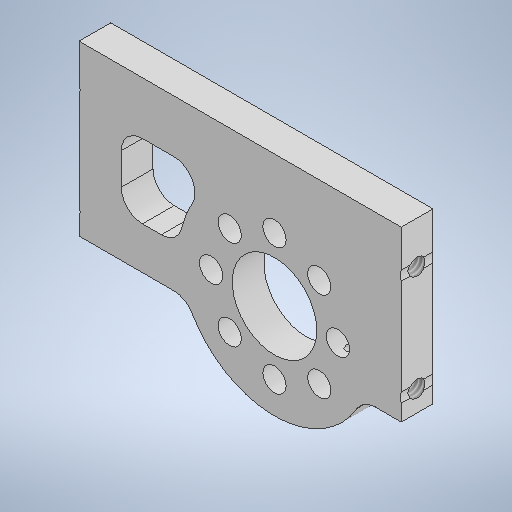
# Autodesk Inventor part: kosipich
Saved by Autodesk Inventor 2025.1 (Build 291241000, 241)
## iProperties
Created: 2024-08-31
Part Number: kosipich
Material: 一般
Document SubType Name: Modeling
Designer: right
Density: 1 g/cm^3
Appearance: 既定
Author: right
Autodesk Inventor part; units mm, degrees
ref_plane "YZ Plane" through (0, 0, 0) normal (1, 0, 0) x (0, 1, 0)
ref_plane "XZ Plane" through (0, 0, 0) normal (0, 1, 0) x (-1, 0, 0)
ref_plane "XY Plane" through (0, 0, 0) normal (0, 0, 1) x (1, 0, 0)
sketch "スケッチ1" plane through (0, 0, 0) normal (0, 0, 1) x (1, 0, 0)
  line L0 (-15.25, -12.5) -> (15.25, -12.5)
  line L1 (15.25, -12.5) -> (15.25, 12.5)
  line L2 (15.25, 12.5) -> (-15.25, 12.5)
  line L3 (-15.25, 12.5) -> (-15.25, -12.5)
  line L4 (-15.25, -12.5) -> (15.25, 12.5) construction
  line L5 (15.25, -12.5) -> (-15.25, 12.5) construction
  line L6 (-16.75, -5) -> (16.75, -5)
  line L7 (16.75, -5) -> (16.75, 5)
  line L8 (16.75, 5) -> (-16.75, 5)
  line L9 (-16.75, 5) -> (-16.75, -5)
  line L10 (-16.75, -5) -> (16.75, 5) construction
  line L11 (16.75, -5) -> (-16.75, 5) construction
  circle A0 centre (-15.25, 6.1) radius 1.1
  line L12 (0, 5) -> (0, 0) construction
  line L13 (-16.75, 0) -> (0, 0) construction
  circle A1 centre (-15.25, -6.1) radius 1.1
  circle A2 centre (15.25, 6.1) radius 1.1
  circle A3 centre (15.25, -6.1) radius 1.1
  point P0 (-15.25, -5)
  point P1 (-15.25, -7.2)
  point P2 (15.25, -7.2)
  point P3 (15.25, -5)
  point P4 (15.25, 5)
  point P5 (15.25, 7.2)
  point P6 (-15.25, 7.2)
  point P7 (-15.25, 5)
  dimension "d0" = 30.5
  dimension "d1" = 25
  dimension "d2" = 1.5
  dimension "d3" = 10
  dimension "d4" = 2.2
  constraints: 28 end point, 6 midpoint, 4 centre point, 4 parallel, 3 symmetric about line, 2 horizontal, 2 perpendicular, 1 point on line, 1 tangent, 1 vertical, 3 other
  measures "d0" distance of L2.end L1.end
  measures "d1" distance of L2.end L0.start
  measures "d2" distance between parallel lines of L3 L9
  measures "d3" distance of L8.end L6.start
  measures "d4" diameter of A0
extrude "押し出し1" add sketch "スケッチ1" along normal blind 3 contours L3 A1 L6 A3 L1 L0 | L3 A1 | A3 L1 | L3 L8 L1 L6 | A0 L3 L2 L1 A2 L8 | L3 A0 | A2 L1 picked at (-15.0909, -5.7696) picked at (14.886, -6.1442) picked at (-15.1684, 6.4575) picked at (14.9092, 6.4667)
sketch "スケッチ3" plane through (0, 0, 3) normal (0, 0, 1) x (1, 0, 0)
  circle A0 centre (3.25, -3.5) radius 4
  circle A1 centre (3.25, -3.5) radius 6 construction
  circle A2 centre (3.25, 2.5) radius 1.1
  circle A3 centre (-0.9926, 0.7426) radius 1.1
  circle A4 centre (-2.75, -3.5) radius 1.1
  circle A5 centre (-0.9926, -7.7426) radius 1.1
  circle A6 centre (3.25, -9.5) radius 1.1
  circle A7 centre (7.4926, -7.7426) radius 1.1
  circle A8 centre (9.25, -3.5) radius 1.1
  circle A9 centre (7.4926, 0.7426) radius 1.1
  line L0 (15.25, -12.5) -> (15.25, 12.5) projected
  line L1 (15.25, 12.5) -> (-15.25, 12.5) projected
  point P0 (15.25, 0)
  point P1 (15.25, 0)
  dimension "d17" = 12
  dimension "d16" = 8
  dimension "d18" = 2.2
  dimension "d21" = 360
  dimension "d45" = 6
  dimension "d46" = 10
  constraints: 9 centre point, 2 coincident, 2 midpoint, 2 vertical alignment, 19 other
  measures "d16" diameter of A0
  measures "d18" diameter of A2
  measures "d45" horizontal distance of point (15.25, 0) A8.centre
  measures "d46" distance from line of L1 A2.centre
extrude "押し出し2" cut sketch "スケッチ3" against normal blind 3
sketch "スケッチ4" plane through (15.25, -12.5, 0) normal (1, 0, 0) x (0, 0, -1)
  line L0 (0, 25) -> (-3, 25) projected
  line L1 (0, 0) -> (0, 25) projected
  point P0 (0, 12.5)
  point P1 (-1.5, 17.5)
  point P2 (-1.5, 7.5)
  point P3 (-1.5, 25)
  point P4 (0, 12.5)
  dimension "d25" = 10
  dimension "d26" = 5
  constraints: 2 midpoint, 2 vertical alignment
  measures "d25" distance of point (-1.5, 7.5) point (-1.5, 17.5)
  measures "d26" vertical distance of point (0, 12.5) point (-1.5, 17.5)
hole "穴2" at (15.25, 5, 1.5) at (15.25, -5, 1.5) direction (-1, 0, 0) diameter 1.567 depth 6.3 tip angle 118 thread size "M2x0.4" class "6H" standard "ISO Metric profile"
sketch "スケッチ5" plane through (-15.25, -12.5, 0) normal (-1, 0, 0) x (0, 0, 1)
  circle A0 centre (1.5, 17.5) radius 0.7835 projected
  circle A1 centre (1.5, 7.5) radius 0.7835 projected
  point P0 (0, 12.5)
  point P1 (2.2448, 17.7431)
  point P2 (0.7552, 17.7431)
  constraints: 2 coincident
hole "穴3" at (-15.25, 5, 1.5) at (-15.25, -5, 1.5) direction (1, 0, 0) diameter 1.567 depth 6.3 tip angle 118 thread size "M2x0.4" class "6H" standard "ISO Metric profile"
sketch "スケッチ6" plane through (0, 0, 3) normal (0, 0, 1) x (1, 0, 0)
  circle A0 centre (-16.25, 5) radius 1.1
  line L0 (-15.25, 4.2165) -> (-15.25, 5.7835) projected
  line L1 (-15.25, -5.7835) -> (-15.25, -4.2165) projected
  line L2 (15.25, 5.7835) -> (15.25, 4.2165) construction
  line L3 (15.25, -4.2165) -> (15.25, -5.7835) construction
  line L4 (-15.25, 12.5) -> (-15.25, -12.5) construction
  line L5 (-15.25, 0) -> (15.25, 0) construction
  line L6 (15.25, -12.5) -> (15.25, 12.5) construction
  line L7 (15.25, 12.5) -> (-15.25, 12.5) construction
  line L8 (0, 12.5) -> (0, 0) construction
  circle A1 centre (-16.25, -5) radius 1.1
  circle A2 centre (16.25, 5) radius 1.1
  circle A3 centre (16.25, -5) radius 1.1
  point P0 (-15.25, 5)
  point P1 (-15.25, 5.4583)
  point P2 (-15.25, 4.5417)
  dimension "d41" = 2.2
  dimension "d42" = 1
  constraints: 4 centre point, 4 end point, 4 midpoint, 3 symmetric about line, 1 horizontal alignment, 1 perpendicular, 3 other
  measures "d41" diameter of A0
  measures "d42" horizontal distance of L0.end A0.centre
extrude "押し出し3" cut sketch "スケッチ6" against normal through all contours A0 L0 | A1 L1 | L1 A1 | A2 | A3 picked at (-15.2316, 4.8964)
sketch "スケッチ7" plane through (0, 0, 3) normal (0, 0, 1) x (1, 0, 0)
  circle A0 centre (3.25, -3.5) radius 4 projected
  circle A1 centre (3.25, -3.5) radius 9
  line L0 (-15.25, -12.5) -> (15.25, -12.5) projected
  line L1 (15.25, -12.5) -> (15.25, -5.4583) projected
  line L2 (15.25, -7) -> (11.5416, -7)
  arc A2 (15.25, -4.5417) -> (15.25, -5.4583) centre (16.25, -5) ccw projected
  line L3 (-5.0416, -7) -> (-15.25, -7)
  line L4 (-15.25, -5.4583) -> (-15.25, -12.5) projected
  line L5 (15.25, 8.9791) -> (-15.25, 8.9791)
  line L6 (-15.25, 12.5) -> (-15.25, 5.4583) projected
  arc A3 (15.25, -4.5417) -> (15.25, -5.4583) centre (16.25, -5) ccw projected
  line L7 (15.25, -4.5417) -> (15.25, 4.5417) projected
  arc A4 (15.25, 5.4583) -> (15.25, 4.5417) centre (16.25, 5) ccw projected
  line L8 (15.25, 5.4583) -> (15.25, 12.5) projected
  line L9 (15.25, 12.5) -> (-15.25, 12.5) projected
  line L10 (-15.25, 12.5) -> (-15.25, 5.4583) projected
  arc A5 (-15.25, 4.5417) -> (-15.25, 5.4583) centre (-16.25, 5) ccw projected
  line L11 (-15.25, 4.5417) -> (-15.25, -4.5417) projected
  arc A6 (-15.25, -5.4583) -> (-15.25, -4.5417) centre (-16.25, -5) ccw projected
  line L12 (-15.25, -5.4583) -> (-15.25, -12.5) projected
  line L13 (-15.25, -12.5) -> (15.25, -12.5) projected
  line L14 (15.25, -12.5) -> (15.25, -5.4583) projected
  circle A7 centre (3.25, -3.5) radius 4 projected
  circle A8 centre (3.25, -9.5) radius 1.1 projected
  circle A9 centre (3.25, 2.5) radius 1.1 projected
  circle A10 centre (-0.9926, -7.7426) radius 1.1 projected
  circle A11 centre (7.4926, 0.7426) radius 1.1 projected
  circle A12 centre (-0.9926, 0.7426) radius 1.1 projected
  circle A13 centre (7.4926, -7.7426) radius 1.1 projected
  circle A14 centre (-2.75, -3.5) radius 1.1 projected
  circle A15 centre (9.25, -3.5) radius 1.1 projected
  line L15 (12.25, -3.5) -> (12.25, 8.9791)
  line L16 (-11.25, -7) -> (-11.25, 8.9791)
  line L17 (-5.7361, -3) -> (-11.25, -3)
  line L18 (-1.7249, 4) -> (-11.25, 4)
  point P0 (0, 0)
  point P1 (15.15, -5)
  point P2 (3.25, -12.5)
  dimension "d47" = 2
  dimension "d51" = 4
  dimension "d53" = 4
  dimension "d54" = 7
  constraints: 14 end point, 7 point on line, 6 point on circle, 4 horizontal, 2 midpoint, 2 perpendicular, 2 tangent, 1 centre point, 1 coincident, 1 horizontal alignment, 1 vertical
  measures "d47" distance from line of point (15.15, -5) L2
  measures "d51" distance between parallel lines of L11 L16
  measures "d53" distance between parallel lines of L3 L17
  measures "d54" distance between parallel lines of L17 L18
extrude "押し出し4" cut sketch "スケッチ7" against normal through all contours A1 L17 L16 L18 | L2 L1 L0 A1 | L5 L6 L9 L8 | L0 L4 L3 A1
fillet "フィレット1" radius 2 2 edges at (11.5416, -7, 1.5) (-5.0416, -7, 1.5)
fillet "フィレット2" radius 2 4 edges at (-11.25, -3, 1.5) (-5.7361, -3, 1.5) (-1.7249, 4, 1.5) (-11.25, 4, 1.5)
